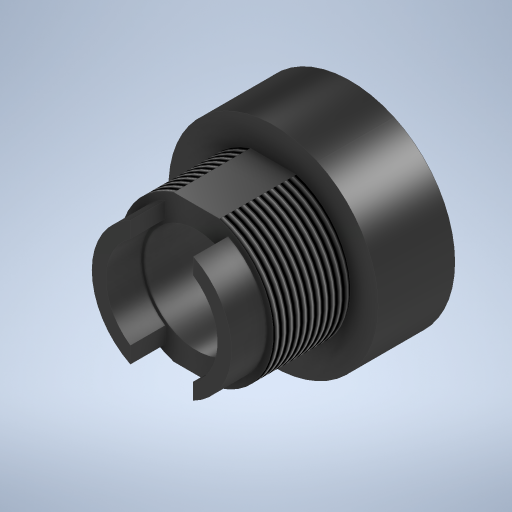
# Autodesk Inventor part: CARCAÇA DO BOTÃO
Saved by Autodesk Inventor 2023 (Build 270158000, 158)
## iProperties
Created: 2023-10-18
Part Number: CARCAÇA DO BOTÃO
Material: Genérico
Document SubType Name: Modeling
Designer: vinicius.sena
Density: 1 g/cm^3
Appearance: Padrão
Author: vinicius.sena
Autodesk Inventor part; units mm, degrees
ref_plane "YZ Plane" through (0, 0, 0) normal (1, 0, 0) x (0, 1, 0)
ref_plane "XZ Plane" through (0, 0, 0) normal (0, 1, 0) x (-1, 0, 0)
ref_plane "XY Plane" through (0, 0, 0) normal (0, 0, 1) x (1, 0, 0)
sketch "Esboço1" plane through (0, 0, 0) normal (0, 0, 1) x (1, 0, 0)
  circle A0 centre (0, 0) radius 12.5
  circle A1 centre (0, 0) radius 15
  dimension "d0" = 25
  dimension "d1" = 30
  constraints: 2 centre point, 2 coincident
  measures "d0" diameter of A0
  measures "d1" diameter of A1
extrude "Extrusão1" add sketch "Esboço1" along normal blind 11
sketch "Esboço2" plane through (0, 0, 11) normal (0, 0, 1) x (1, 0, 0)
  circle A0 centre (0, 0) radius 15
  dimension "d4" = 30
  constraints: 1 centre point, 1 coincident
  measures "d4" diameter of A0
extrude "Extrusão2" add sketch "Esboço2" against normal blind 3
sketch "Esboço4" plane through (0, 0, 11) normal (0, 0, 1) x (1, 0, 0)
  circle A0 centre (0, 0) radius 11
  dimension "d10" = 22
  constraints: 1 centre point, 1 coincident
  measures "d10" diameter of A0
extrude "Extrusão4" add sketch "Esboço4" along normal blind 16
sketch "Esboço5" plane through (0, 0, 27) normal (0, 0, 1) x (1, 0, 0)
  circle A0 centre (0, 0) radius 7.5
  dimension "d13" = 15
  constraints: 1 centre point, 1 coincident
  measures "d13" diameter of A0
extrude "Extrusão5" cut sketch "Esboço5" against normal through all
sketch "Esboço6" plane through (0, 0, 27) normal (0, 0, 1) x (1, 0, 0)
  circle A0 centre (0, 0) radius 10
  circle A1 centre (0, 0) radius 8
  circle A2 centre (0, 0) radius 7.5
  circle A3 centre (0, 0) radius 11
  dimension "d16" = 20
  dimension "d27" = 16
  dimension "d28" = 22
  constraints: 4 centre point, 3 coincident
  measures "d16" diameter of A0
  measures "d27" diameter of A1
  measures "d28" diameter of A3
extrude "Extrusão6" cut sketch "Esboço6" against normal blind 5
thread "Rosca1" size "M22x1" class "6g" standard "ANSI Metric M Profile" length 15
sketch "Esboço7" plane through (0, 0, 0) normal (0, 1, 0) x (-1, 0, 0)
  line L0 (4.5, 22) -> (-4.5, 22)
  line L1 (-4.5, 22) -> (-4.5, 27)
  line L2 (-4.5, 27) -> (4.5, 27)
  line L3 (4.5, 27) -> (4.5, 22)
  line L4 (4.5, 22) -> (-4.5, 27) construction
  line L5 (-4.5, 22) -> (4.5, 27) construction
  line L6 (10, 27) -> (-10, 27) projected
  point P0 (0, 0)
  point P1 (0, 24.5)
  dimension "d22" = 9
  dimension "d23" = 5
  dimension "d24" = 0
  constraints: 12 end point, 2 midpoint, 2 parallel, 1 horizontal, 1 perpendicular
  measures "d22" distance of L1.end L2.end
  measures "d23" distance of L0.end L1.end
  measures "d24" distance between parallel lines of L6 L2
extrude "Extrusão7" cut sketch "Esboço7" along normal through all both and the other way through all
sketch "Esboço8" plane through (0, 0, 22) normal (0, 0, 1) x (1, 0, 0)
  line L0 (-10.5, 10.5) -> (10.5, 10.5)
  line L1 (10.5, 10.5) -> (10.5, -10.5)
  line L2 (10.5, -10.5) -> (-10.5, -10.5)
  line L3 (-10.5, -10.5) -> (-10.5, 10.5)
  line L4 (-10.5, 10.5) -> (10.5, -10.5) construction
  line L5 (10.5, 10.5) -> (-10.5, -10.5) construction
  circle A0 centre (0, 0) radius 11
  point P0 (-3.2787, -10.5)
  point P1 (3.2787, -10.5)
  point P2 (3.2787, 10.5)
  point P3 (-3.2787, 10.5)
  dimension "d29" = 21
  dimension "d30" = 21
  dimension "d31" = 22
  constraints: 12 end point, 2 midpoint, 2 parallel, 1 centre point, 1 coincident, 1 horizontal, 1 perpendicular
  measures "d29" distance of L1.end L2.end
  measures "d30" distance of L0.end L1.end
  measures "d31" diameter of A0
extrude "Extrusão8" cut sketch "Esboço8" against normal blind 11 contours A0 L0 | L2 A0
